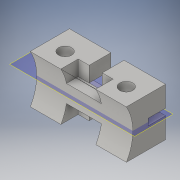
# Autodesk Inventor part: back_pack_clip_in_2
Saved by Autodesk Inventor 2016 (Build 200138000, 138)
## iProperties
Created: 2016-05-05
Part Number: back_pack_clip_in_2
Material: Generic
Document SubType Name: Modeling
Designer: ajar021
Density: 1 g/cm^3
Appearance: Default
Author: ajar021
Autodesk Inventor part; units mm, degrees
ref_plane "YZ Plane" through (0, 0, 0) normal (1, 0, 0) x (0, 1, 0)
ref_plane "XZ Plane" through (0, 0, 0) normal (0, 1, 0) x (-1, 0, 0)
ref_plane "XY Plane" through (0, 0, 0) normal (0, 0, 1) x (1, 0, 0)
sketch "Sketch1" plane through (0, 0, 0) normal (0, 0, 1) x (1, 0, 0)
  line L0 (-11, 5.5) -> (11, 5.5)
  line L1 (11, 5.5) -> (11, -5.5)
  line L2 (11, -5.5) -> (-11, -5.5)
  line L3 (-11, -5.5) -> (-11, 5.5)
  line L4 (-11, 5.5) -> (11, -5.5) construction
  line L5 (11, 5.5) -> (-11, -5.5) construction
  point P0 (0, 0)
  dimension "d0" = 22
  dimension "d1" = 11
  constraints: 12 end point, 2 midpoint, 2 parallel, 1 horizontal, 1 perpendicular
  measures "d0" distance of L0.start L0.end
  measures "d1" distance of L2.end L0.start
extrude "Extrusion1" add sketch "Sketch1" along normal blind 9
sketch "Sketch2" plane through (-11, 5.5, 0) normal (0, 1, 0) x (1, 0, 0)
  line L0 (0, 0) -> (0, -9) projected
  line L1 (22, 0) -> (22, -9) projected
  circle A0 centre (4, -5) radius 1.5
  circle A1 centre (18, -5) radius 1.5
  line L2 (0, 0) -> (22, 0) projected
  line L3 (22, 0) -> (22, -9) projected
  line L4 (4, 0) -> (4, -5)
  line L5 (18, -5) -> (18, 0)
  line L6 (0, -5) -> (4, -5)
  line L7 (22, -5) -> (18, -5)
  point P0 (11, 0)
  point P1 (9, -4)
  dimension "d6" = 3
  dimension "d7" = 3
  dimension "d25" = 5
  dimension "d26" = 5
  dimension "d27" = 4
  dimension "d28" = 4
  constraints: 8 end point, 4 point on line, 3 perpendicular, 2 centre point, 1 vertical
  measures "d6" diameter of A0
  measures "d7" diameter of A1
  measures "d25" distance of L4.start L4.end
  measures "d26" distance of L5.start L5.end
  measures "d27" distance of L6.start L4.end
  measures "d28" distance of L7.start L5.start
extrude "Extrusion2" cut sketch "Sketch2" against normal up to next contours L6 L4 A0 | A0 L4 L6 | L5 L7 A1 | A1 L7 L5
sketch "Sketch3" plane through (11, -5.5, 0) normal (1, 0, 0) x (0, 0, -1)
  line L0 (-9, 0) -> (-9, 11) projected
  line L1 (0, 0) -> (-9, 0) projected
  line L2 (-9, 11) -> (-9, 0)
  line L3 (-9, 11) -> (-9, 0) projected
  arc A0 (-9, -0.0647) -> (-9, 11) centre (-18.452, 5.4676) ccw
  line L4 (-9, 11) -> (-9, -0.0647)
  line L5 (-6.5, 11) -> (-6.5, 0) projected
  line L6 (0, 0) -> (0, 11) projected
  line L7 (0, 6.25) -> (0, 4.75)
  point P0 (0, 5.5)
  constraints: 6 end point, 2 collinear, 2 point on circle, 2 point on line, 1 centre point
extrude "Extrusion3" cut sketch "Sketch3" against normal up to next
sketch "Sketch6" plane through (0, 0, 0) normal (0, 0, -1) x (-1, 0, 0)
  line L0 (-11, 5.5) -> (-11, -5.5) projected
  line L1 (-11, 5.5) -> (-11, 2.5)
  line L2 (-11, -5.5) -> (11, -5.5) projected
  line L3 (-11, -5.5) -> (-11, -2.5)
  line L4 (0, 0) -> (0, -2)
  line L5 (0, -2) -> (9, -2)
  line L6 (0, 0) -> (0, 2)
  line L7 (0, 2) -> (-9, 2)
  line L8 (9, -2) -> (-9, -2)
  line L9 (-9, -2) -> (-9, 2)
  line L10 (-9, 2) -> (9, 2)
  line L11 (9, 2) -> (9, -2)
  line L12 (-11, -5.5) -> (11, -5.5) projected
  line L13 (11, -5.5) -> (11, 5.5) projected
  dimension "d40" = 2
  dimension "d41" = 9
  dimension "d42" = 2
  dimension "d43" = 9
  constraints: 20 end point, 3 perpendicular, 2 parallel, 2 point on line, 2 vertical, 1 horizontal
  measures "d40" distance of L4.start L4.end
  measures "d41" distance of L4.end L5.end
  measures "d42" distance of L4.start L6.end
  measures "d43" distance of L6.end L7.end
extrude "Extrusion6" cut sketch "Sketch6" against normal blind 5
sketch "Sketch4" plane through (-11, -5.5, 0) normal (0, -1, 0) x (1, 0, 0)
  line L0 (11, 0) -> (11, 2.5)
  line L1 (0, 0) -> (22, 0) projected
  line L2 (12.5, 5) -> (9.5, 5)
  line L3 (9.5, 5) -> (9.5, 0)
  line L4 (9.5, 0) -> (12.5, 0)
  line L5 (12.5, 0) -> (12.5, 5)
  line L6 (12.5, 5) -> (9.5, 0) construction
  line L7 (9.5, 5) -> (12.5, 0) construction
  line L8 (22, 8.9624) -> (0, 8.9624) projected
  line L9 (12.5, 5) -> (15, 5)
  line L10 (15, 5) -> (15, 8.9624)
  line L11 (9.5, 5) -> (7, 5)
  line L12 (7, 5) -> (7, 9)
  line L13 (22, 9) -> (0, 9) projected
  line L14 (7, 9) -> (15, 8.9624)
  dimension "d13" = 2.5
  dimension "d14" = 3
  dimension "d34" = 2.5
  dimension "d35" = 2.5
  constraints: 24 end point, 4 point on line, 3 perpendicular, 2 horizontal, 2 midpoint, 2 parallel, 1 vertical
  measures "d13" distance of L0.start L0.end
  measures "d14" distance of L4.end L3.end
  measures "d34" distance of L2.start L9.end
  measures "d35" distance of L2.end L11.end
extrude "Extrusion4" cut sketch "Sketch4" against normal up to surface (3.5 mm away)
sketch "Sketch5" plane through (11, -5.5, 0) normal (1, 0, 0) x (0, 0, -1)
  line L0 (0, 5.5) -> (-4, 5.5)
  line L1 (-5, 0) -> (-5, 3) projected
  line L2 (0, 5.5) -> (0, 4.75)
  line L3 (0, 0) -> (0, 11) projected
  line L4 (-4, 5.5) -> (-4, 6.25)
  line L5 (0, 4.75) -> (-4, 4.75)
  line L6 (-4, 4.75) -> (-4, 6.25)
  line L7 (-4, 6.25) -> (0, 6.25)
  line L8 (0, 6.25) -> (0, 4.75)
  point P0 (-5, 11)
  dimension "d20" = 4
  dimension "d21" = 0.75
  dimension "d22" = 0.75
  constraints: 14 end point, 2 parallel, 2 perpendicular, 1 horizontal, 1 point on line, 1 vertical
  measures "d20" distance of L0.start L0.end
  measures "d21" distance of L0.start L2.end
  measures "d22" distance of L0.end L4.end
extrude "Extrusion5" cut sketch "Sketch5" against normal up to next
ref_plane "Work Plane1" through (11, 0, 0) normal (0, -1, 0) x (1, 0, 0)
mirror "Mirror1" about plane through (11, 0, 0) normal (0, -1, 0) of "Extrusion4"
equation "\"d7\" = d6"
equation "\"d26\" = d25"
equation "\"d28\" = d27"
equation "\"d22\" = d21"
body "Solid1"
